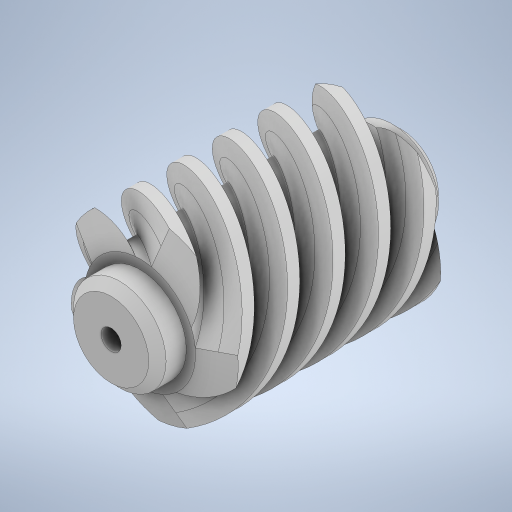
# Autodesk Inventor part: sens_fi_final_2
Saved by Autodesk Inventor 2024.2 (Build 282272000, 272)
## iProperties
Created: 2024-03-04
Part Number: sens_fi_final_2
Material: Genérico
Document SubType Name: Modeling
Designer: riera
Density: 1 g/cm^3
Appearance: Valor por defecto
Author: riera
Autodesk Inventor part; units mm, degrees
ref_plane "YZ Plane" through (0, 0, 0) normal (1, 0, 0) x (0, 1, 0)
ref_plane "XZ Plane" through (0, 0, 0) normal (0, 1, 0) x (-1, 0, 0)
ref_plane "XY Plane" through (0, 0, 0) normal (0, 0, 1) x (1, 0, 0)
sketch "Boceto1" plane through (0, 0, 0) normal (0, 0, 1) x (1, 0, 0)
  circle A0 centre (0, 0) radius 30
  dimension "d0" = 60
  constraints: 1 centre point, 1 coincident
  measures "d0" diameter of A0
extrude "Extrusión1" add sketch "Boceto1" along normal mid plane 80.111
sketch "Boceto2" plane through (0, 0, 40.0555) normal (0, 0, 1) x (1, 0, 0)
  circle A0 centre (0, 0) radius 25
  dimension "d3" = 50
  constraints: 1 centre point, 1 coincident
  measures "d3" diameter of A0
surface extrude "diametre separacio" sketch "Boceto2" against normal blind 80.111 shown no curves A0
chamfer "Chaflán1" distance 10.835 distance2 3.944 1 edges at (-30, 0, 40.0555) measured on face at (-29.5, 0, 40.0555)
chamfer "Chaflán2" distance 10.835 distance2 3.944 1 edges at (-30, 0, -40.0555) measured on face at (-29.5, 0, -40.0555)
sketch "Boceto3" plane through (0, 0, 0) normal (1, 0, 0) x (0, 1, 0)
  line L0 (30, 60.7249) -> (30, 49.2311)
  line L1 (30, 49.2311) -> (19.165, 53.1748)
  line L2 (19.165, 53.1748) -> (19.165, 56.7812)
  line L3 (19.165, 56.7812) -> (30, 60.7249)
  line L4 (25, 54.978) -> (25, 51.051)
  point P0 (0, 0)
  point P1 (30, 54.978)
  point P2 (30, 54.978)
  point P3 (19.165, 54.978)
  dimension "d12" = 54.978
  dimension "d13" = 110
  dimension "d14" = 30
  dimension "d15" = 19.165
  dimension "d16" = 25
  dimension "d17" = 3.927
  constraints: 10 end point, 2 horizontal alignment, 2 midpoint, 2 vertical, 1 coincident, 1 parallel, 1 point on line
  measures "d12" vertical distance of point (0, 0) point (30, 54.978)
  measures "d13" angle of L2 L3
  measures "d14" distance from line of point (0, 0) L0
  measures "d15" distance from line of point (0, 0) L2
  measures "d16" horizontal distance of point (0, 0) L4.start
  measures "d17" distance of L4.start L4.end
coil "Bobina1" sketch "Boceto3" operation cut axis through (0, 0, -10) along (0, 0, -1) pitch 78.54 turns 8 hand left
pattern_circular "Patrón circular1" count 5 over 360 about axis through (0, 0, -10) along (0, 0, 1) of "Bobina1"
sketch "Boceto4" plane through (0, 0, 40.0555) normal (0, 0, 1) x (1, 0, 0)
  circle A0 centre (0, 0) radius 16
  dimension "d29" = 32
  constraints: 1 centre point, 1 coincident
  measures "d29" diameter of A0
extrude "Extrusión2" add sketch "Boceto4" along normal blind 10
chamfer "Chaflán3" distance 3 angle 45 1 edges at (-16, 0, 50.0555) measured on face at (-15.5, 0, 50.0555)
mirror "Simetría1" about plane through (0, 0, 0) normal (0, 0, 1) of "Extrusión2", "Chaflán3"
sketch "Boceto5" plane through (0, 0, 50.0555) normal (0, 0, 1) x (1, 0, 0)
  circle A0 centre (0, 0) radius 13 projected
  circle A1 centre (0, 0) radius 3.5
  dimension "d35" = 7
  constraints: 1 centre point, 1 coincident
  measures "d35" diameter of A1
extrude "Extrusión3" cut sketch "Boceto5" against normal through all contours A1
